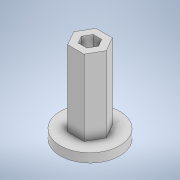
# Autodesk Inventor part: 5mm.125in insert
Saved by Autodesk Inventor 2020 (Build 240168000, 168)
## iProperties
Created: 2019-12-30
Part Number: 5mm.125in insert
Material: Generic
Document SubType Name: Modeling
Designer: xj82b
Density: 1 g/cm^3
Appearance: Default
Author: xj82b
Autodesk Inventor part; units mm, degrees
ref_plane "YZ Plane" through (0, 0, 0) normal (1, 0, 0) x (0, 1, 0)
ref_plane "XZ Plane" through (0, 0, 0) normal (0, 1, 0) x (-1, 0, 0)
ref_plane "XY Plane" through (0, 0, 0) normal (0, 0, 1) x (1, 0, 0)
sketch "Sketch1" plane through (0, 0, 0) normal (0, 1, 0) x (-1, 0, 0)
  line L0 (2.7496, -4.7625) -> (-2.7496, -4.7625)
  line L1 (-2.7496, -4.7625) -> (-5.4993, 0)
  line L2 (-5.4993, 0) -> (-2.7496, 4.7625)
  line L3 (-2.7496, 4.7625) -> (2.7496, 4.7625)
  line L4 (2.7496, 4.7625) -> (5.4993, 0)
  line L5 (5.4993, 0) -> (2.7496, -4.7625)
  line L6 (1.4434, -2.5) -> (-1.4434, -2.5)
  line L7 (-1.4434, -2.5) -> (-2.8868, 0)
  line L8 (-2.8868, 0) -> (-1.4434, 2.5)
  line L9 (-1.4434, 2.5) -> (1.4434, 2.5)
  line L10 (1.4434, 2.5) -> (2.8868, 0)
  line L11 (2.8868, 0) -> (1.4434, -2.5)
  point P0 (0, 0)
  point P1 (0, 0)
  point P2 (0, 0)
  dimension "d0" = 9.525
  dimension "d1" = 5
  constraints: 24 end point, 2 coincident, 2 horizontal, 26 other
  measures "d0" distance between parallel lines of L4 L1
  measures "d1" distance between parallel lines of L8 L11
extrude "Extrusion1" add sketch "Sketch1" along normal blind 25.4
sketch "Sketch2" plane through (0, 0, 0) normal (0, -1, 0) x (1, 0, 0)
  line L0 (1.4434, -2.5) -> (-1.4434, -2.5)
  line L1 (-1.4434, -2.5) -> (-2.8868, 0)
  line L2 (-2.8868, 0) -> (-1.4434, 2.5)
  line L3 (-1.4434, 2.5) -> (1.4434, 2.5)
  line L4 (1.4434, 2.5) -> (2.8868, 0)
  line L5 (2.8868, 0) -> (1.4434, -2.5)
  line L6 (1.4434, -2.5) -> (2.8868, 0) projected
  circle A0 centre (0, 0) radius 10
  dimension "d4" = 20
  constraints: 12 end point, 2 coincident, 1 centre point, 1 equal length, 1 horizontal, 13 other
  measures "d4" diameter of A0
extrude "Extrusion2" add sketch "Sketch2" along normal blind 3
body "Solid1"
